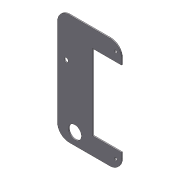
# Autodesk Inventor part: Plate_VerticalConveyorMotorMount
Saved by Autodesk Inventor 2012 (Build 160160000, 160)
## iProperties
Created: 2012-02-25
Part Number: Plate_VerticalConveyorMotorMount
Material: Aluminum-6061
Document SubType Name: Modeling
Designer: JesseK
Density: 2.71 g/cm^3
Mass: 141.299 g
Surface Area: 461.852 cm^2
Volume: 52.14 cm^3
Author: JesseK
Autodesk Inventor part; units mm, degrees
ref_plane "YZ Plane" through (0, 0, 0) normal (1, 0, 0) x (0, 1, 0)
ref_plane "XZ Plane" through (0, 0, 0) normal (0, 1, 0) x (-1, 0, 0)
ref_plane "XY Plane" through (0, 0, 0) normal (0, 0, 1) x (1, 0, 0)
sketch "Sketch1" plane through (0, 0, 0) normal (0, 0, 1) x (1, 0, 0)
  line L0 (0, 0) -> (139.7, 0)
  line L1 (139.7, 241.3) -> (0, 241.3)
  line L2 (0, 241.3) -> (0, 0)
  line L3 (139.7, 203.2) -> (76.2, 203.2)
  line L4 (76.2, 203.2) -> (76.2, 38.1)
  line L5 (76.2, 38.1) -> (139.7, 38.1)
  line L6 (139.7, 0) -> (139.7, 38.1)
  line L7 (139.7, 203.2) -> (139.7, 241.3)
  circle A0 centre (127, 222.25) radius 3.175
  circle A1 centre (127, 19.05) radius 3.175
  circle A2 centre (19.05, 139.7) radius 4.7625
  circle A3 centre (38.1, 25.4) radius 14.2875
  dimension "d0" = 38.1
  dimension "d1" = 38.1
  dimension "d2" = 241.3
  dimension "d3" = 139.7
  dimension "d4" = 12.7
  dimension "d5" = 12.7
  dimension "d6" = 6.35
  dimension "d7" = 6.35
  dimension "d8" = 19.05
  dimension "d9" = 19.05
  dimension "d10" = 63.5
  dimension "d11" = 9.525
  dimension "d12" = 19.05
  dimension "d13" = 101.6
  dimension "d14" = 28.575
  dimension "d15" = 38.1
  dimension "d16" = 25.4
  constraints: 16 end point, 4 centre point, 4 parallel, 3 perpendicular, 2 horizontal, 1 collinear
  measures "d0" distance of L3.start L1.start
  measures "d1" distance of L0.end L5.end
  measures "d2" distance of L1.end L0.start
  measures "d3" distance of L0.start L0.end
  measures "d4" distance from line of L6 A1.centre
  measures "d5" distance from line of L7 A0.centre
  measures "d6" diameter of A0
  measures "d7" diameter of A1
  measures "d8" distance from line of L0 A1.centre
  measures "d9" distance from line of L1 A0.centre
  measures "d10" distance of L3.start L3.end
  measures "d11" diameter of A2
  measures "d12" distance from line of L2 A2.centre
  measures "d13" distance from line of L1 A2.centre
  measures "d14" diameter of A3
  measures "d15" distance from line of L2 A3.centre
  measures "d16" distance from line of L0 A3.centre
extrude "Extrusion1" add sketch "Sketch1" along normal blind 2.3813
fillet "Fillet1" radius 25.4 4 edges at (0, 241.3, 1.1906) (139.7, 241.3, 1.1906) (0, 0, 1.1906) (139.7, 0, 1.1906)
body "Solid1"
